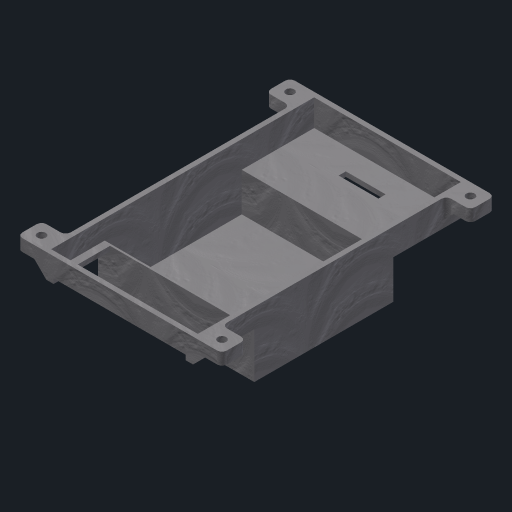
# Autodesk Inventor part: CAJA_P1
Saved by Autodesk Inventor 2024.3 (Build 283343000, 343)
## iProperties
Created: 2024-07-22
Part Number: CAJA_P1
Material: Steel, Mild, Welded
Document SubType Name: Modeling
Designer: Niler
Density: 7.85 g/cm^3
Appearance: Weld - Steel Mild
Author: Niler
Autodesk Inventor part; units mm, degrees
ref_plane "YZ Plane" through (0, 0, 0) normal (1, 0, 0) x (0, 1, 0)
ref_plane "XZ Plane" through (0, 0, 0) normal (0, 1, 0) x (-1, 0, 0)
ref_plane "XY Plane" through (0, 0, 0) normal (0, 0, 1) x (1, 0, 0)
sketch "Sketch1" plane through (0, 0, 0) normal (0, 1, 0) x (-1, 0, 0)
  line L0 (-30, 54.1) -> (30, 54.1)
  line L1 (30, 54.1) -> (30, -54.1)
  line L2 (30, -54.1) -> (-30, -54.1)
  line L3 (-30, -54.1) -> (-30, 54.1)
  line L4 (-30, 54.1) -> (30, -54.1) construction
  line L5 (30, 54.1) -> (-30, -54.1) construction
  line L6 (30.4, -54.5) -> (30.4, 54.5)
  line L7 (30.4, 54.5) -> (-30.4, 54.5)
  line L8 (-30.4, 54.5) -> (-30.4, -54.5)
  line L9 (-30.4, -54.5) -> (30.4, -54.5)
  line L10 (32.4, 56.5) -> (32.4, -56.5)
  line L11 (32.4, -56.5) -> (-32.4, -56.5)
  line L12 (-32.4, -56.5) -> (-32.4, 56.5)
  line L13 (-32.4, 56.5) -> (32.4, 56.5)
  point P0 (0, 0)
  dimension "d0" = 60
  dimension "d1" = 108.2
  dimension "d2" = 0.4
  dimension "d3" = 2
  constraints: 28 end point, 6 parallel, 3 perpendicular, 2 midpoint, 1 horizontal, 6 other
  measures "d0" distance of L1.end L2.end
  measures "d1" distance of L0.end L1.end
  measures "d2" distance between parallel lines of L1 L6
  measures "d3" distance between parallel lines of L6 L10
extrude "Extrusion1" add sketch "Sketch1" along normal blind 27 contours L10 L11 L12 L13
extrude "Extrusion2" add sketch "Sketch1" against normal blind 2 contours L0 L1 L2 L3 | L9 L8 L7 L6 | L10 L11 L12 L13
sketch "Sketch2" plane through (0, -2, 0) normal (0, -1, 0) x (1, 0, 0)
  line L0 (32.4, -56.5) -> (32.4, 56.5) projected
  line L1 (32.4, 56.5) -> (-32.4, 56.5) projected
  line L2 (-32.4, 56.5) -> (-32.4, -56.5) projected
  line L3 (-32.4, -56.5) -> (32.4, -56.5) projected
  line L4 (-32.4, -24.5) -> (32.4, -24.5)
  point P0 (0, 0)
  dimension "d8" = 32
  constraints: 2 end point, 2 point on line, 1 perpendicular
  measures "d8" distance between parallel lines of L4 L3
extrude "Extrusion3" cut sketch "Sketch2" against normal blind 18 contours L3 L2 L4 L0
sketch "Sketch3" plane through (0, 16, 0) normal (0, -1, 0) x (1, 0, 0)
  line L0 (-30.4, -24.5) -> (-30.4, -54.5) projected
  line L1 (-32.4, -24.5) -> (-30.4, -24.5) projected
  line L2 (-32.4, -56.5) -> (-32.4, -24.5) projected
  line L3 (32.4, -56.5) -> (-32.4, -56.5) projected
  line L4 (32.4, -24.5) -> (32.4, -56.5) projected
  line L5 (30.4, -24.5) -> (32.4, -24.5) projected
  line L6 (30.4, -54.5) -> (30.4, -24.5) projected
  line L7 (-30.4, -54.5) -> (30.4, -54.5) projected
  line L8 (-30.4, -24.5) -> (30.4, -24.5)
  point P0 (0, 0)
  constraints: 2 end point, 1 collinear
extrude "Extrusion4" add sketch "Sketch3" along normal blind 2
sketch "Sketch4" plane through (0, 14, 0) normal (0, -1, 0) x (1, 0, 0)
  line L0 (-32.4, -24.5) -> (-32.4, -56.5) projected
  line L1 (-32.4, -56.5) -> (32.4, -56.5) projected
  line L2 (32.4, -56.5) -> (32.4, -24.5) projected
  line L3 (30.4, -24.5) -> (32.4, -24.5) projected
  line L4 (30.4, -24.5) -> (-30.4, -24.5) projected
  line L5 (-32.4, -24.5) -> (-30.4, -24.5) projected
  line L6 (-32.4, -26.5) -> (32.4, -26.5)
  point P0 (0, 0)
  dimension "d13" = 2
  constraints: 2 end point, 2 point on line, 1 perpendicular
  measures "d13" distance between parallel lines of L6 L4
extrude "Extrusion5" add sketch "Sketch4" along normal up to surface (16 mm away) contours L5 L4 L3 L2 L6 L0
sketch "Sketch5" plane through (0, 14, 0) normal (0, -1, 0) x (1, 0, 0)
  line L0 (32.4, -26.5) -> (-32.4, -26.5) projected
  line L1 (-32.4, -26.5) -> (-32.4, -56.5) projected
  line L2 (-32.4, -56.5) -> (32.4, -56.5) projected
  line L3 (32.4, -56.5) -> (32.4, -26.5) projected
  line L4 (8.25, -45.5) -> (-8.25, -45.5)
  line L5 (-8.25, -45.5) -> (-8.25, -42.5)
  line L6 (-8.25, -42.5) -> (8.25, -42.5)
  line L7 (8.25, -42.5) -> (8.25, -45.5)
  line L8 (8.25, -45.5) -> (-8.25, -42.5) construction
  line L9 (-8.25, -45.5) -> (8.25, -42.5) construction
  point P0 (0, 0)
  point P1 (0, -44)
  point P2 (0, -56.5)
  dimension "d16" = 16.5
  dimension "d18" = 14
  dimension "d19" = 3
  constraints: 12 end point, 3 midpoint, 2 parallel, 1 horizontal, 1 perpendicular, 1 vertical alignment
  measures "d16" distance of L5.end L6.end
  measures "d18" distance between parallel lines of L6 L2
  measures "d19" distance of L6.end L4.start
extrude "Extrusion6" cut sketch "Sketch5" against normal through all contours L4 L5 L6 L7
sketch "Sketch7" plane through (0, -2, 0) normal (0, -1, 0) x (1, 0, 0)
  line L0 (32.4, -26.5) -> (32.4, 56.5) projected
  line L1 (32.4, 56.5) -> (-32.4, 56.5) projected
  line L2 (-32.4, -26.5) -> (-32.4, 56.5) projected
  line L3 (32.4, -26.5) -> (-32.4, -26.5) projected
  line L4 (-32.4, 32.3) -> (32.4, 32.3)
  point P0 (0, 0)
  dimension "d25" = 24.2
  constraints: 2 end point, 2 point on line, 1 perpendicular
  measures "d25" distance between parallel lines of L1 L4
extrude "Extrusion7" cut sketch "Sketch7" against normal blind 21 contours L4 L2 L1 L0
sketch "Sketch8" plane through (0, 19, 0) normal (0, -1, 0) x (1, 0, 0)
  line L0 (-30.4, 54.5) -> (-30.4, 32.3) projected
  line L1 (30.4, 54.5) -> (-30.4, 54.5) projected
  line L2 (30.4, 32.3) -> (30.4, 54.5) projected
  line L3 (32.4, 32.3) -> (30.4, 32.3) projected
  line L4 (32.4, 56.5) -> (32.4, 32.3) projected
  line L5 (-32.4, 56.5) -> (32.4, 56.5) projected
  line L6 (-32.4, 32.3) -> (-32.4, 56.5) projected
  line L7 (-30.4, 32.3) -> (-32.4, 32.3) projected
  line L8 (32.4, 32.3) -> (30.4, 32.3) projected
  line L9 (30.4, 32.3) -> (-30.4, 32.3)
  line L10 (-32.4, 32.3) -> (-32.4, 56.5) projected
  line L11 (-32.4, 33.1) -> (32.4, 33.1)
  point P0 (0, 0)
  dimension "d28" = 0.8
  constraints: 4 end point, 2 point on line, 1 collinear, 1 perpendicular
  measures "d28" distance between parallel lines of L11 L9
extrude "Extrusion8" add sketch "Sketch8" along normal blind 21 contours L11 L2 L9 L0 | L0 L7 L6 L11 | L11 L4 L3 L2
sketch "Sketch9" plane through (0, 19, 0) normal (0, -1, 0) x (1, 0, 0)
  line L0 (30.4, 33.1) -> (32.4, 33.1) projected
  line L1 (32.4, 56.5) -> (32.4, 33.1) projected
  line L2 (-32.4, 56.5) -> (32.4, 56.5) projected
  line L3 (-32.4, 33.1) -> (-32.4, 56.5) projected
  line L4 (-32.4, 33.1) -> (-30.4, 33.1) projected
  line L5 (-30.4, 54.5) -> (-30.4, 33.1) projected
  line L6 (30.4, 54.5) -> (-30.4, 54.5) projected
  line L7 (30.4, 33.1) -> (30.4, 54.5) projected
  line L8 (30.4, 33.1) -> (30.4, 54.5) projected
  line L9 (30.4, 54.5) -> (-30.4, 54.5) projected
  line L10 (30.4, 33.1) -> (27.4, 33.1)
  line L11 (27.4, 33.1) -> (27.4, 54.5)
  line L12 (27.4, 54.5) -> (30.4, 54.5)
  line L13 (30.4, 54.5) -> (30.4, 33.1)
  line L14 (-30.4, 54.5) -> (-27.4, 54.5)
  line L15 (-27.4, 54.5) -> (-27.4, 33.1)
  line L16 (-27.4, 33.1) -> (-30.4, 33.1)
  line L17 (-30.4, 33.1) -> (-30.4, 54.5)
  line L18 (27.4, 54.5) -> (27.4, 56.5)
  line L19 (-30.4, 54.5) -> (-30.4, 33.1) projected
  line L20 (-30.4, 54.5) -> (-30.4, 56.5)
  line L21 (-27.4, 54.5) -> (-27.4, 56.5)
  point P0 (0, 0)
  dimension "d31" = 3
  dimension "d32" = 3
  constraints: 22 end point, 6 point on line, 4 parallel, 4 perpendicular, 2 horizontal
  measures "d31" distance between parallel lines of L5 L15
  measures "d32" distance between parallel lines of L7 L11
extrude "Extrusion9" add sketch "Sketch9" along normal blind 2 contours L7 L6 L18 L2 L1 L0 | L10 L11 L6 L7 | L15 L16 L5 L6 | L6 L20 L2 L21 | L5 L4 L3 L2 L20
sketch "Sketch11" plane through (0, 27, 0) normal (0, 1, 0) x (1, 0, 0)
  line L0 (32.4, -56.5) -> (32.4, 56.5) projected
  line L1 (32.4, 56.5) -> (-32.4, 56.5) projected
  line L2 (-32.4, 56.5) -> (-32.4, -56.5) projected
  line L3 (-32.4, -56.5) -> (32.4, -56.5) projected
  line L4 (-30.4, 54.5) -> (30.4, 54.5) projected
  line L5 (30.4, 54.5) -> (30.4, -54.5) projected
  line L6 (30.4, -54.5) -> (-30.4, -54.5) projected
  line L7 (-30.4, -54.5) -> (-30.4, 54.5) projected
  line L8 (-32.4, -56.5) -> (-42.4, -56.5)
  line L9 (-42.4, -56.5) -> (-42.4, -46.5)
  line L10 (-42.4, -46.5) -> (-32.4, -46.5)
  line L11 (-32.4, -46.5) -> (-32.4, -56.5)
  line L12 (0, 0) -> (-16.3575, 0)
  line L13 (-16.3575, 0) -> (0, 0)
  line L14 (0, 0) -> (0, -19.6836)
  circle A0 centre (-37.4, -51.5) radius 1.75
  line L15 (-32.4, 56.5) -> (-42.4, 56.5)
  line L16 (-42.4, 56.5) -> (-42.4, 46.5)
  line L17 (-42.4, 46.5) -> (-32.4, 46.5)
  line L18 (-32.4, 46.5) -> (-32.4, 56.5)
  circle A1 centre (-37.4, 51.5) radius 1.75
  line L19 (32.4, -56.5) -> (42.4, -56.5)
  line L20 (42.4, -56.5) -> (42.4, -46.5)
  line L21 (42.4, -46.5) -> (32.4, -46.5)
  line L22 (32.4, -46.5) -> (32.4, -56.5)
  circle A2 centre (37.4, -51.5) radius 1.75
  line L23 (32.4, 46.5) -> (32.4, 56.5)
  line L24 (32.4, 56.5) -> (42.4, 56.5)
  line L25 (42.4, 46.5) -> (32.4, 46.5)
  line L26 (42.4, 56.5) -> (42.4, 46.5)
  circle A3 centre (37.4, 51.5) radius 1.75
  point P0 (-37.4, -46.5)
  point P1 (-42.4, -51.5)
  point P2 (-37.4, 46.5)
  point P3 (-42.4, 51.5)
  point P4 (37.4, -46.5)
  point P5 (42.4, -51.5)
  point P6 (37.4, 46.5)
  point P7 (42.4, 51.5)
  dimension "d40" = 3.5
  dimension "d41" = 10
  dimension "d42" = 10
  constraints: 38 end point, 18 symmetric about line, 4 centre point, 3 equal length, 2 horizontal, 2 midpoint, 1 horizontal alignment, 1 perpendicular, 1 vertical, 1 vertical alignment, 3 other
  measures "d40" diameter of A0
  measures "d41" distance of L8.end L9.end
  measures "d42" distance of L2.end L8.end
extrude "Extrusion11" add sketch "Sketch11" against normal blind 5 contours L0 L21 L20 L19 | L8 L9 L10 L2 | L0 L24 L26 L25 | L17 L16 L15 L2
chamfer "Chamfer2" distance 3 angle 45 4 edges at (-32.4, 22, 51.5) (32.4, 22, 51.5) (32.4, 22, -51.5) (-32.4, 22, -51.5)
sketch "Sketch12" plane through (0, 22, 0) normal (0, -1, 0) x (1, 0, 0)
  circle A0 centre (-37.4, -51.5) radius 1.75 projected
  circle A1 centre (-37.4, 51.5) radius 1.75 projected
  circle A2 centre (37.4, 51.5) radius 1.75 projected
  circle A3 centre (37.4, -51.5) radius 1.75 projected
  circle A4 centre (37.4, -51.5) radius 2.9
  circle A5 centre (37.4, 51.5) radius 2.9
  circle A6 centre (-37.4, 51.5) radius 2.9
  circle A7 centre (-37.4, -51.5) radius 2.9
  point P0 (0, 0)
  dimension "d48" = 5.8
  constraints: 4 centre point, 4 coincident, 3 equal radius
  measures "d48" diameter of A4
extrude "Extrusion12" cut sketch "Sketch12" along normal mid plane 6 contours A2 | A4 | A5 | A6 | A7
fillet "Fillet1" radius 2 12 edges at (42.4, 24.5, -56.5) (42.4, 24.5, -46.5) (42.4, 24.5, 46.5) (42.4, 24.5, 56.5) (32.4, 23, 46.5) (32.4, 23, -46.5) (-42.4, 24.5, 56.5) (-42.4, 24.5, 46.5) (-32.4, 23, 46.5) (-32.4, 23, -46.5) (-42.4, 24.5, -46.5) (-42.4, 24.5, -56.5)
chamfer "Chamfer3" distance 2 angle 45 6 edges at (-32.4, -2, 3.3) (32.4, -2, 3.3) (32.4, 14, -41.5) (-32.4, 14, -41.5) (32.4, 17, 44.8) (-32.4, 17, 44.8)
chamfer "Chamfer4" distance 2 angle 45 8 edges at (0, -2, -26.5) (0, -2, 33.1) (0, 14, -56.5) (0, 14, -26.5) (-32.4, 15, -26.5) (-32.4, 7, -26.5) (32.4, 6.9999, -26.5) (32.4, 15, -26.5)
body "Solid1"
